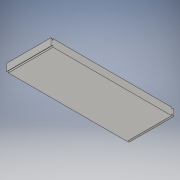
# Autodesk Inventor part: doveTailBar
Saved by Autodesk Inventor 2016 (Build 200138000, 138)
## iProperties
Created: 2015-11-04
Part Number: doveTailBar
Material: Generic
Document SubType Name: Modeling
Designer: rossmosier
Density: 1 g/cm^3
Appearance: Default
Author: rossmosier
Autodesk Inventor part; units mm, degrees
ref_plane "YZ Plane" through (0, 0, 0) normal (1, 0, 0) x (0, 1, 0)
ref_plane "XZ Plane" through (0, 0, 0) normal (0, 1, 0) x (-1, 0, 0)
ref_plane "XY Plane" through (0, 0, 0) normal (0, 0, 1) x (1, 0, 0)
sketch "Sketch1" plane through (0, 0, 0) normal (0, 1, 0) x (-1, 0, 0)
  line L0 (0, 0) -> (-209.55, 0)
  line L1 (-209.55, 0) -> (-209.55, 12.7)
  line L2 (-209.55, 12.7) -> (0, 12.7)
  line L3 (0, 12.7) -> (0, 0)
  line L4 (0, 12.7) -> (-3.302, 12.7) construction
  line L5 (-3.302, 12.7) -> (-3.302, 0) construction
  line L6 (-3.302, 12.7) -> (-3.302, 9.652) construction
  line L7 (-3.302, 0) -> (-3.302, 3.048) construction
  line L8 (0, 6.35) -> (0, 0.254) construction
  line L9 (0, 6.35) -> (0, 12.446) construction
  line L10 (0, 12.446) -> (-3.302, 9.652)
  line L11 (0, 0.254) -> (-3.302, 3.048)
  line L12 (-3.302, 3.048) -> (-3.302, 9.652)
  line L13 (-3.302, 9.652) -> (-3.302, 12.7)
  line L14 (-3.302, 3.048) -> (-3.302, 0)
  line L15 (-104.775, 0) -> (-104.775, 12.7) construction
  line L16 (-209.55, 12.7) -> (-209.55, 0)
  line L17 (-209.55, 6.35) -> (-209.55, 0.254) construction
  line L18 (-209.55, 6.35) -> (-209.55, 12.446) construction
  line L19 (-209.55, 12.446) -> (-206.248, 9.652)
  line L20 (-209.55, 0.254) -> (-206.248, 3.048)
  line L21 (-206.248, 3.048) -> (-206.248, 9.652)
  line L22 (-206.248, 9.652) -> (-206.248, 12.7)
  line L23 (-206.248, 3.048) -> (-206.248, 0)
  dimension "d0" = 209.55
  dimension "d1" = 12.7
  dimension "d2" = 3.302
  dimension "d3" = 3.048
  dimension "d4" = 3.048
  dimension "d5" = 6.096
  dimension "d6" = 6.096
  constraints: 48 end point, 11 point on line, 5 symmetric about line, 3 collinear, 3 midpoint, 3 perpendicular, 2 parallel, 1 horizontal
  measures "d0" distance of L1.end L2.end
  measures "d1" distance of L0.end L1.end
  measures "d2" distance of L2.end L4.end
  measures "d3" distance of L4.end L6.end
  measures "d4" distance of L5.end L7.end
  measures "d5" distance of L8.start L8.end
  measures "d6" distance of L8.start L9.end
extrude "Extrusion1" add sketch "Sketch1" along normal blind 76.2 contours L0 L23 L21 L22 L2 L13 L12 L14 | L11 L12 L10 L3 | L20 L1 L19 L21
body "Solid1"
